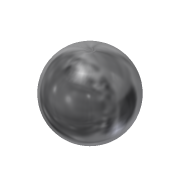
# Autodesk Inventor part: m3 6
Saved by Autodesk Inventor 2014 (Build 180170000, 170)
## iProperties
Created: 2016-03-31
Part Number: m3 6
Material: Steel
Document SubType Name: Modeling
Designer: admin
Density: 7.85 g/cm^3
Appearance: Steel Galvanized
Author: admin
Autodesk Inventor part; units mm, degrees
ref_plane "YZ Plane" through (0, 0, 0) normal (1, 0, 0) x (0, 1, 0)
ref_plane "XZ Plane" through (0, 0, 0) normal (0, 1, 0) x (-1, 0, 0)
ref_plane "XY Plane" through (0, 0, 0) normal (0, 0, 1) x (1, 0, 0)
sketch "Sketch5" plane through (0, 0, 0) normal (0, 1, 0) x (-1, 0, 0)
  arc A0 (0, 5) -> (-2.7129, -4.2) centre (0, 0) ccw
  line L0 (-2.7129, -4.2) -> (0, -4.2)
  line L1 (0, 5) -> (0, -4.2)
  dimension "d15" = 10
  dimension "d16" = 9.2
  constraints: 4 end point, 2 point on circle, 1 centre point, 1 coincident, 1 horizontal
  measures "d15" diameter of A0
revolve "Revolution1" add sketch "Sketch5" angle 360 about axis through (0, 0, 5) along (0, 0, -1)
sketch "Sketch6" plane through (0, 0, -4.2) normal (0, 0, -1) x (-1, 0, 0)
  circle A0 centre (0, 0) radius 2.7129 projected
hole "Hole1" at (0, 0, -4.2) direction (0, 0, 1) diameter 3.242 depth 7 tip angle 118 thread size "M4x0.7" class "6H" standard "ISO Metric profile"
chamfer "Chamfer1" distance 0.3 angle 45 1 edges at (0, -1.621, -4.2)
body "Solid2"
